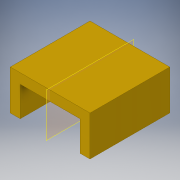
# Autodesk Inventor part: WIREBRIDGE
Saved by Autodesk Inventor 2017 (Build 210142000, 142)
## iProperties
Created: 2018-01-06
Part Number: WIREBRIDGE
Material: ABS Plastic
Document SubType Name: Modeling
Designer: Delta
Density: 1.06 g/cm^3
Appearance: Gold
Author: Delta
Autodesk Inventor part; units mm, degrees
ref_plane "YZ Plane" through (0, 0, 0) normal (1, 0, 0) x (0, 1, 0)
ref_plane "XZ Plane" through (0, 0, 0) normal (0, 1, 0) x (-1, 0, 0)
ref_plane "XY Plane" through (0, 0, 0) normal (0, 0, 1) x (1, 0, 0)
sketch "Sketch1" plane through (0, 0, 0) normal (0, 1, 0) x (-1, 0, 0)
  point P0 (0, 0)
sketch "Sketch2" plane through (0, 0, 0) normal (0, 0, 1) x (1, 0, 0)
  line L0 (0, 0) -> (50.8, 0)
  line L1 (50.8, 0) -> (50.8, 25.4)
  line L2 (50.8, 25.4) -> (0, 25.4)
  line L3 (0, 25.4) -> (0, 0)
  line L4 (6.35, 0) -> (44.45, 0)
  line L5 (44.45, 0) -> (44.45, 19.05)
  line L6 (44.45, 19.05) -> (6.35, 19.05)
  line L7 (6.35, 19.05) -> (6.35, 0)
  dimension "d0" = 6.35
  dimension "d1" = 6.35
  dimension "d2" = 6.35
  dimension "d3" = 38.1
  dimension "d4" = 25.4
  constraints: 16 end point, 4 parallel, 2 horizontal, 2 perpendicular, 1 point on line
  measures "d0" distance between parallel lines of L3 L7
  measures "d1" distance between parallel lines of L2 L6
  measures "d2" distance between parallel lines of L1 L5
  measures "d3" distance of L5.end L6.end
  measures "d4" distance between parallel lines of L0 L2
extrude "Extrusion1" add sketch "Sketch2" along normal blind 50.8 contours L3 L2 L1 L0 L5 L6 L7
ref_plane "Work Plane1" through (25.4, 0, 0) normal (1, 0, 0) x (0, 0, -1)
sketch "Sketch4" plane through (0, 0, 0) normal (0, -1, 0) x (1, 0, 0)
  circle A0 centre (3.175, 44.45) radius 1.651
  line L0 (6.35, 0) -> (6.35, 50.8) projected
  line L1 (0, 50.8) -> (6.35, 50.8) projected
  circle A1 centre (3.175, 6.35) radius 1.651
  line L2 (0, 0) -> (6.35, 0) projected
  line L3 (50.8, 50.8) -> (0, 50.8) projected
  line L4 (25.4, 50.8) -> (25.4, 0)
  line L5 (50.8, 0) -> (0, 0) projected
  circle A2 centre (47.625, 44.45) radius 1.651
  circle A3 centre (47.625, 6.35) radius 1.651
  dimension "d13" = 3.302
  dimension "d14" = 3.175
  dimension "d15" = 6.35
  dimension "d16" = 3.302
  dimension "d17" = 6.35
  constraints: 4 centre point, 2 end point, 2 midpoint, 2 symmetric about line, 2 other
  measures "d13" diameter of A0
  measures "d14" distance from line of L0 A0.centre
  measures "d15" distance from line of L1 A0.centre
  measures "d16" diameter of A1
  measures "d17" distance from line of L2 A1.centre
extrude "Extrusion2" cut sketch "Sketch4" against normal blind 12.7 contours A0 | A1 | A2 | A3
body "Solid1"
